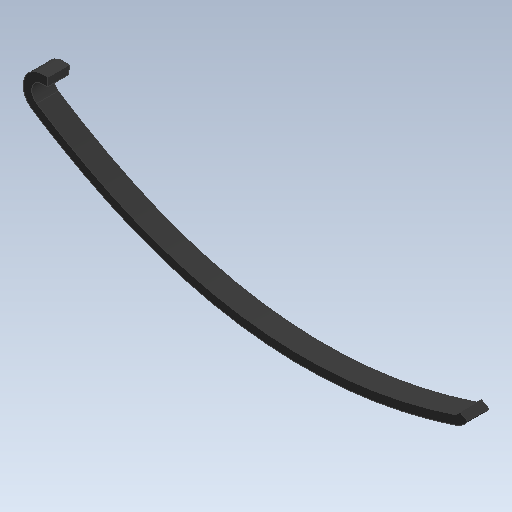
# Autodesk Inventor part: 脚ゴム
Saved by Autodesk Inventor 2020.2 (Build 242310000, 310)
## iProperties
Created: 2020-03-29
Part Number: 脚ゴム
Material: ゴム、シリコーン
Document SubType Name: Modeling
Designer: aoyama
Density: 1.25 g/cm^3
Appearance: ゴム - 黒
Mass: 1.4401 g
Surface Area: 16.3295 cm^2
Volume: 1.15208 cm^3
Author: aoyama
Autodesk Inventor part; units mm, degrees
ref_plane "YZ Plane" through (0, 0, 0) normal (1, 0, 0) x (0, 1, 0)
ref_plane "XZ Plane" through (0, 0, 0) normal (0, 1, 0) x (-1, 0, 0)
ref_plane "XY Plane" through (0, 0, 0) normal (0, 0, 1) x (1, 0, 0)
sketch "スケッチ1" plane through (0, 0, 0) normal (0, 0, 1) x (1, 0, 0)
  circle A0 centre (0, -30) radius 22.5
  arc A1 (33.5221, -76.1381) -> (34.7879, -75.2018) centre (32.744, -73.7622) ccw
  arc A2 (25.323, -41.3574) -> (34.2025, -71.7318) centre (49.1917, -50.8648) ccw
  arc A3 (25.323, -41.3574) -> (17.6049, -10.4152) centre (-0.0473, -31.252) ccw
  arc A4 (17.6049, -10.4152) -> (7.2408, -4.7162) centre (-0.2944, -30.6931) ccw
  arc A5 (5.1078, -1.4883) -> (7.2408, -4.7162) centre (8.0549, -1.8596) ccw
  arc A6 (5.1078, -1.4883) -> (-5.8369, -1.4852) centre (-0.3643, -0.7018) ccw
  arc A7 (-5.8369, -1.4852) -> (-5.7215, -2.051) centre (-0.3936, -0.6703) ccw
  arc A8 (-7.4636, -3.4089) -> (-5.7215, -2.051) centre (-8.3074, -0.53) ccw
  arc A9 (-7.4636, -3.4089) -> (-26.8108, -27.5489) centre (0.1311, -29.3188) ccw
  arc A10 (-61.6776, -57.4439) -> (-26.8108, -27.5489) centre (-58.8657, -25.4432) ccw
  arc A11 (-61.6776, -57.4439) -> (-63.2531, -62.0341) centre (-61.8964, -59.9343) ccw
  spline S0 degree 4 poles (-63.2531, -62.0341) (-62.8771, -62.2771) (-62.3536, -62.6129) (-61.6848, -63.0378) (-60.873, -63.5467) (-60.2895, -63.9093) (-59.7104, -64.266) (-59.1355, -64.6169) (-58.5645, -64.9622) (-57.9972, -65.3021) (-57.4335, -65.6368) (-56.873, -65.9663) (-56.3156, -66.2909) (-55.7612, -66.6107) (-55.2095, -66.9258) (-54.6604, -67.2364) (-54.1137, -67.5424) (-53.5693, -67.8442) (-53.027, -68.1416) (-52.4867, -68.4349) (-51.9483, -68.7242) (-51.4116, -69.0094) (-50.8766, -69.2907) (-50.3432, -69.5682) (-49.8111, -69.8419) (-49.2804, -70.1119) (-48.7509, -70.3783) (-48.2225, -70.6411) (-47.6953, -70.9003) (-47.169, -71.156) (-46.6436, -71.4083) (-46.119, -71.6572) (-45.5953, -71.9028) (-45.0722, -72.145) (-44.5498, -72.384) (-44.0279, -72.6197) (-43.5066, -72.8522) (-42.9857, -73.0816) (-42.4653, -73.3077) (-41.9453, -73.5308) (-41.4255, -73.7507) (-40.9061, -73.9676) (-40.3869, -74.1814) (-39.868, -74.3922) (-39.3492, -74.5999) (-38.8305, -74.8047) (-38.312, -75.0064) (-37.7935, -75.2052) (-37.2751, -75.401) (-36.7567, -75.5939) (-36.2383, -75.7839) (-35.7198, -75.9709) (-35.2014, -76.155) (-34.6828, -76.3362) (-34.1642, -76.5146) (-33.6454, -76.69) (-33.1265, -76.8625) (-32.6075, -77.0322) (-32.0883, -77.199) (-31.5689, -77.363) (-31.0494, -77.5241) (-30.5297, -77.6823) (-30.0097, -77.8377) (-29.4895, -77.9902) (-28.9692, -78.1399) (-28.4485, -78.2868) (-27.9276, -78.4308) (-27.4065, -78.572) (-26.8851, -78.7103) (-26.3635, -78.8459) (-25.8416, -78.9785) (-25.3194, -79.1084) (-24.797, -79.2354) (-24.2743, -79.3596) (-23.7513, -79.481) (-23.228, -79.5995) (-22.7044, -79.7153) (-22.1806, -79.8281) (-21.6564, -79.9382) (-21.132, -80.0454) (-20.6073, -80.1498) (-20.0824, -80.2514) (-19.5571, -80.3501) (-19.0316, -80.446) (-18.5058, -80.5391) (-17.9797, -80.6294) (-17.4533, -80.7168) (-16.9267, -80.8014) (-16.3998, -80.8831) (-15.8727, -80.962) (-15.3453, -81.0381) (-14.8176, -81.1114) (-14.2897, -81.1818) (-13.7615, -81.2494) (-13.2331, -81.3141) (-12.7045, -81.376) (-12.1756, -81.4351) (-11.6464, -81.4913) (-11.1171, -81.5447) (-10.5875, -81.5953) (-10.0577, -81.643) (-9.5277, -81.6879) (-8.9975, -81.7299) (-8.467, -81.7691) (-7.9364, -81.8055) (-7.4055, -81.839) (-6.8745, -81.8697) (-6.3432, -81.8975) (-5.8118, -81.9225) (-5.2802, -81.9447) (-4.7483, -81.964) (-4.2163, -81.9805) (-3.6842, -81.9941) (-3.1518, -82.005) (-2.6192, -82.0129) (-2.0865, -82.0181) (-1.5536, -82.0204) (-1.0205, -82.0198) (-0.4873, -82.0165) (0.0461, -82.0103) (0.5798, -82.0012) (1.1136, -81.9893) (1.6475, -81.9746) (2.1817, -81.9571) (2.716, -81.9367) (3.2506, -81.9135) (3.7853, -81.8874) (4.3203, -81.8585) (4.8554, -81.8268) (5.3907, -81.7923) (5.9263, -81.7549) (6.4621, -81.7146) (6.9982, -81.6716) (7.5345, -81.6257) (8.071, -81.5769) (8.6078, -81.5254) (9.1449, -81.4709) (9.6823, -81.4137) (10.22, -81.3536) (10.758, -81.2906) (11.2964, -81.2248) (11.8351, -81.1561) (12.3742, -81.0846) (12.9137, -81.0102) (13.4537, -80.933) (13.9941, -80.8528) (14.5349, -80.7698) (15.0763, -80.6839) (15.6182, -80.5952) (16.1606, -80.5035) (16.7036, -80.4089) (17.2473, -80.3114) (17.7916, -80.211) (18.3366, -80.1077) (18.8824, -80.0014) (19.4289, -79.8921) (19.9763, -79.7799) (20.5245, -79.6647) (21.0736, -79.5465) (21.6238, -79.4253) (22.1749, -79.301) (22.7271, -79.1737) (23.2805, -79.0433) (23.835, -78.9099) (24.3908, -78.7733) (24.948, -78.6336) (25.5066, -78.4907) (26.0666, -78.3446) (26.6283, -78.1953) (27.1915, -78.0427) (27.7565, -77.8868) (28.3233, -77.7276) (28.8921, -77.5651) (29.4629, -77.3991) (30.0358, -77.2297) (30.6109, -77.0568) (31.1884, -76.8803) (31.9873, -76.6323) (32.6434, -76.4238) (33.1553, -76.2582) (33.5221, -76.1381) knots 0 0 0 0 0 0.015592 0.021777 0.027929 0.034049 0.040138 0.046199 0.052232 0.058238 0.064219 0.070176 0.076109 0.08202 0.08791 0.093779 0.099629 0.105459 0.111272 0.117067 0.122846 0.128609 0.134356 0.140089 0.145808 0.151513 0.157206 0.162886 0.168554 0.17421 0.179856 0.185491 0.191116 0.196731 0.202337 0.207934 0.213522 0.219102 0.224675 0.230239 0.235796 0.241346 0.246889 0.252426 0.257957 0.263481 0.269 0.274513 0.280021 0.285523 0.291021 0.296514 0.302002 0.307486 0.312966 0.318442 0.323914 0.329382 0.334846 0.340307 0.345765 0.351219 0.356671 0.362119 0.367565 0.373008 0.378448 0.383886 0.389321 0.394754 0.400185 0.405614 0.41104 0.416465 0.421888 0.427309 0.432729 0.438147 0.443563 0.448978 0.454391 0.459803 0.465214 0.470624 0.476032 0.48144 0.486846 0.492252 0.497656 0.50306 0.508463 0.513865 0.519267 0.524668 0.530069 0.535469 0.540869 0.546268 0.551667 0.557066 0.562465 0.567863 0.573262 0.57866 0.584059 0.589457 0.594856 0.600255 0.605655 0.611054 0.616454 0.621855 0.627256 0.632658 0.63806 0.643464 0.648868 0.654273 0.659678 0.665086 0.670494 0.675903 0.681314 0.686726 0.69214 0.697555 0.702972 0.708391 0.713811 0.719234 0.724659 0.730086 0.735515 0.740947 0.746382 0.751819 0.757259 0.762702 0.768149 0.773599 0.779052 0.784509 0.789969 0.795434 0.800903 0.806376 0.811854 0.817337 0.822825 0.828317 0.833816 0.83932 0.84483 0.850346 0.855869 0.861399 0.866935 0.872479 0.878031 0.883591 0.889159 0.894736 0.900321 0.905917 0.911522 0.917137 0.922763 0.9284 0.934049 0.93971 0.945383 0.951069 0.956769 0.962483 0.968212 0.973956 0.979716 0.985493 1 1 1 1 1
  arc A12 (34.1445, -78.0387) -> (35.3693, -70.1074) centre (32.744, -73.7622) ccw
  arc A13 (27.181, -42.0975) -> (35.3693, -70.1074) centre (49.1917, -50.8648) ccw
  arc A14 (27.181, -42.0975) -> (18.9132, -8.9024) centre (-0.0473, -31.252) ccw
  arc A15 (18.9132, -8.9024) -> (7.7922, -2.7937) centre (-0.2944, -30.6931) ccw
  arc A16 (7.0908, -1.7497) -> (7.7922, -2.7937) centre (8.0549, -1.8596) ccw
  arc A17 (7.0908, -1.7497) -> (-7.8158, -1.7749) centre (-0.3643, -0.7018) ccw
  arc A18 (-7.8158, -1.7749) -> (-7.8596, -1.4241) centre (-0.3936, -0.6703) ccw
  arc A19 (-8.0261, -1.4896) -> (-7.8596, -1.4241) centre (-8.3074, -0.53) ccw
  arc A20 (-8.0261, -1.4896) -> (-28.8065, -27.4178) centre (0.1311, -29.3188) ccw
  arc A21 (-61.5025, -55.4515) -> (-28.8065, -27.4178) centre (-58.8657, -25.4432) ccw
  arc A22 (-61.5025, -55.4515) -> (-64.3384, -63.714) centre (-61.8964, -59.9343) ccw
  line L0 (32.744, -73.7622) -> (36.7043, -75.899)
  line L1 (-58.8657, -25.4432) -> (-60.8013, -57.5088)
  line L2 (-61.8964, -59.9343) -> (-65.1475, -63.0456)
  line L3 (-61.8964, -59.9343) -> (-65.7346, -57.5851)
  line L4 (49.1917, -50.8648) -> (30.5824, -70.5938)
  arc A23 (-5.8375, -1.4811) -> (-5.8362, -1.4893) centre (-4.7979, -1.3331) ccw
  arc A24 (-5.8362, -1.4893) -> (-5.8121, -1.6365) centre (-0.3936, -0.6703) ccw
  arc A25 (-6.0587, -2.5158) -> (-5.8121, -1.6365) centre (-6.8458, -1.8208) ccw
  arc A26 (-7.4636, -3.4089) -> (-6.0587, -2.5158) centre (-8.3074, -0.53) ccw
  arc A27 (-7.4636, -3.4089) -> (-26.8108, -27.5489) centre (0.1311, -29.3188) ccw
  arc A28 (-61.6776, -57.4439) -> (-26.8108, -27.5489) centre (-58.8657, -25.4432) ccw
  arc A29 (-61.6776, -57.4439) -> (-63.2531, -62.0341) centre (-61.8964, -59.9343) ccw
  spline S1 degree 4 poles (-63.2531, -62.0341) (-62.8771, -62.2771) (-62.3536, -62.6129) (-61.6848, -63.0378) (-60.873, -63.5467) (-60.2895, -63.9093) (-59.7104, -64.266) (-59.1355, -64.6169) (-58.5645, -64.9622) (-57.9972, -65.3021) (-57.4335, -65.6368) (-56.873, -65.9663) (-56.3156, -66.2909) (-55.7612, -66.6107) (-55.2095, -66.9258) (-54.6604, -67.2364) (-54.1137, -67.5424) (-53.5693, -67.8442) (-53.027, -68.1416) (-52.4867, -68.4349) (-51.9483, -68.7242) (-51.4116, -69.0094) (-50.8766, -69.2907) (-50.3432, -69.5682) (-49.8111, -69.8419) (-49.2804, -70.1119) (-48.7509, -70.3783) (-48.2225, -70.6411) (-47.6953, -70.9003) (-47.169, -71.156) (-46.6436, -71.4083) (-46.119, -71.6572) (-45.5953, -71.9028) (-45.0722, -72.145) (-44.5498, -72.384) (-44.0279, -72.6197) (-43.5066, -72.8522) (-42.9857, -73.0816) (-42.4653, -73.3077) (-41.9453, -73.5308) (-41.4255, -73.7507) (-40.9061, -73.9676) (-40.3869, -74.1814) (-39.868, -74.3922) (-39.3492, -74.5999) (-38.8305, -74.8047) (-38.312, -75.0064) (-37.7935, -75.2052) (-37.2751, -75.401) (-36.7567, -75.5939) (-36.2383, -75.7839) (-35.7198, -75.9709) (-35.2014, -76.155) (-34.6828, -76.3362) (-34.1642, -76.5146) (-33.6454, -76.69) (-33.1265, -76.8625) (-32.6075, -77.0322) (-32.0883, -77.199) (-31.5689, -77.363) (-31.0494, -77.5241) (-30.5297, -77.6823) (-30.0097, -77.8377) (-29.4895, -77.9902) (-28.9692, -78.1399) (-28.4485, -78.2868) (-27.9276, -78.4308) (-27.4065, -78.572) (-26.8851, -78.7103) (-26.3635, -78.8459) (-25.8416, -78.9785) (-25.3194, -79.1084) (-24.797, -79.2354) (-24.2743, -79.3596) (-23.7513, -79.481) (-23.228, -79.5995) (-22.7044, -79.7153) (-22.1806, -79.8281) (-21.6564, -79.9382) (-21.132, -80.0454) (-20.6073, -80.1498) (-20.0824, -80.2514) (-19.5571, -80.3501) (-19.0316, -80.446) (-18.5058, -80.5391) (-17.9797, -80.6294) (-17.4533, -80.7168) (-16.9267, -80.8014) (-16.3998, -80.8831) (-15.8727, -80.962) (-15.3453, -81.0381) (-14.8176, -81.1114) (-14.2897, -81.1818) (-13.7615, -81.2494) (-13.2331, -81.3141) (-12.7045, -81.376) (-12.1756, -81.4351) (-11.6464, -81.4913) (-11.1171, -81.5447) (-10.5875, -81.5953) (-10.0577, -81.643) (-9.5277, -81.6879) (-8.9975, -81.7299) (-8.467, -81.7691) (-7.9364, -81.8055) (-7.4055, -81.839) (-6.8745, -81.8697) (-6.3432, -81.8975) (-5.8118, -81.9225) (-5.2802, -81.9447) (-4.7483, -81.964) (-4.2163, -81.9805) (-3.6842, -81.9941) (-3.1518, -82.005) (-2.6192, -82.0129) (-2.0865, -82.0181) (-1.5536, -82.0204) (-1.0205, -82.0198) (-0.4873, -82.0165) (0.0461, -82.0103) (0.5798, -82.0012) (1.1136, -81.9893) (1.6475, -81.9746) (2.1817, -81.9571) (2.716, -81.9367) (3.2506, -81.9135) (3.7853, -81.8874) (4.3203, -81.8585) (4.8554, -81.8268) (5.3907, -81.7923) (5.9263, -81.7549) (6.4621, -81.7146) (6.9982, -81.6716) (7.5345, -81.6257) (8.071, -81.5769) (8.6078, -81.5254) (9.1449, -81.4709) (9.6823, -81.4137) (10.22, -81.3536) (10.758, -81.2906) (11.2964, -81.2248) (11.8351, -81.1561) (12.3742, -81.0846) (12.9137, -81.0102) (13.4537, -80.933) (13.9941, -80.8528) (14.5349, -80.7698) (15.0763, -80.6839) (15.6182, -80.5952) (16.1606, -80.5035) (16.7036, -80.4089) (17.2473, -80.3114) (17.7916, -80.211) (18.3366, -80.1077) (18.8824, -80.0014) (19.4289, -79.8921) (19.9763, -79.7799) (20.5245, -79.6647) (21.0736, -79.5465) (21.6238, -79.4253) (22.1749, -79.301) (22.7271, -79.1737) (23.2805, -79.0433) (23.835, -78.9099) (24.3908, -78.7733) (24.948, -78.6336) (25.5066, -78.4907) (26.0666, -78.3446) (26.6283, -78.1953) (27.1915, -78.0427) (27.7565, -77.8868) (28.3233, -77.7276) (28.8921, -77.5651) (29.4629, -77.3991) (30.0358, -77.2297) (30.6109, -77.0568) (31.1884, -76.8803) (31.9873, -76.6323) (32.6434, -76.4238) (33.1553, -76.2582) (33.5221, -76.1381) knots 0 0 0 0 0 0.015592 0.021777 0.027929 0.034049 0.040138 0.046199 0.052232 0.058238 0.064219 0.070176 0.076109 0.08202 0.08791 0.093779 0.099629 0.105459 0.111272 0.117067 0.122846 0.128609 0.134356 0.140089 0.145808 0.151513 0.157206 0.162886 0.168554 0.17421 0.179856 0.185491 0.191116 0.196731 0.202337 0.207934 0.213522 0.219102 0.224675 0.230239 0.235796 0.241346 0.246889 0.252426 0.257957 0.263481 0.269 0.274513 0.280021 0.285523 0.291021 0.296514 0.302002 0.307486 0.312966 0.318442 0.323914 0.329382 0.334846 0.340307 0.345765 0.351219 0.356671 0.362119 0.367565 0.373008 0.378448 0.383886 0.389321 0.394754 0.400185 0.405614 0.41104 0.416465 0.421888 0.427309 0.432729 0.438147 0.443563 0.448978 0.454391 0.459803 0.465214 0.470624 0.476032 0.48144 0.486846 0.492252 0.497656 0.50306 0.508463 0.513865 0.519267 0.524668 0.530069 0.535469 0.540869 0.546268 0.551667 0.557066 0.562465 0.567863 0.573262 0.57866 0.584059 0.589457 0.594856 0.600255 0.605655 0.611054 0.616454 0.621855 0.627256 0.632658 0.63806 0.643464 0.648868 0.654273 0.659678 0.665086 0.670494 0.675903 0.681314 0.686726 0.69214 0.697555 0.702972 0.708391 0.713811 0.719234 0.724659 0.730086 0.735515 0.740947 0.746382 0.751819 0.757259 0.762702 0.768149 0.773599 0.779052 0.784509 0.789969 0.795434 0.800903 0.806376 0.811854 0.817337 0.822825 0.828317 0.833816 0.83932 0.84483 0.850346 0.855869 0.861399 0.866935 0.872479 0.878031 0.883591 0.889159 0.894736 0.900321 0.905917 0.911522 0.917137 0.922763 0.9284 0.934049 0.93971 0.945383 0.951069 0.956769 0.962483 0.968212 0.973956 0.979716 0.985493 1 1 1 1 1
  arc A30 (33.5221, -76.1381) -> (34.7879, -75.2018) centre (32.744, -73.7622) ccw
  arc A31 (34.7879, -75.2018) -> (34.2598, -73.0105) centre (33.5615, -74.3381) ccw
  arc A32 (25.323, -41.3574) -> (30.5824, -70.5938) centre (44.8156, -52.9421) ccw
  arc A33 (25.323, -41.3574) -> (17.6049, -10.4152) centre (-0.0473, -31.252) ccw
  arc A34 (17.6049, -10.4152) -> (7.2408, -4.7162) centre (-0.2944, -30.6931) ccw
  arc A35 (5.1078, -1.4883) -> (7.2408, -4.7162) centre (8.0549, -1.8596) ccw
  arc A36 (5.1078, -1.4883) -> (-5.8375, -1.4811) centre (-0.3643, -0.7018) ccw
  circle A37 centre (0, -30) radius 22.7
  arc A38 (30.5824, -70.5938) -> (34.2598, -73.0105) centre (44.8156, -52.9421) ccw
  arc A39 (34.7879, -75.2018) -> (34.2025, -71.7318) centre (32.744, -73.7622) ccw
  arc A40 (31.8378, -69.0369) -> (35.1909, -71.2404) centre (44.8156, -52.9421) ccw
  arc A41 (36.423, -76.3535) -> (35.1909, -71.2404) centre (33.5615, -74.3381) ccw
  spline S2 degree 5 poles (-64.3384, -63.714) (-58.3884, -67.5577) (-52.2614, -71.1261) (-45.9065, -74.3086) (-33.0908, -79.5522) (-19.6141, -82.7098) (-12.9369, -83.7013) (0.6571, -84.5608) (14.2099, -83.176) (20.9822, -81.9204) (27.6266, -80.1731) (34.1445, -78.0387) knots 0 0 0 0 0 0 0.342867 0.342867 0.342867 0.668023 0.668023 0.668023 1 1 1 1 1 1
  point P0 (0, 0)
  point P1 (0, 0)
  point P2 (34.9441, -74.9493)
  point P3 (-60.6808, -55.5124)
  point P4 (-63.7026, -61.6628)
  point P5 (-64.0288, -58.6292)
  point P6 (32.9348, -68.0999)
  point P7 (0, 0)
  point P8 (-5.8121, -1.6365)
  point P9 (25.323, -41.3574)
  point P10 (-5.8121, -1.6365)
  point P11 (34.9441, -74.9493)
  point P12 (-63.7026, -61.6628)
  point P13 (25.323, -41.3574)
  point P14 (36.6963, -75.8947)
  point P15 (31.9593, -69.1341)
  point P16 (34.9338, -74.9438)
  dimension "d0" = 2
  dimension "d3" = 2
  constraints: 84 point on circle, 42 centre point, 10 end point, 1 concentric, 1 line through centre, 59 other
  measures "d3" radial gap between concentric circles of A40 A38
extrude "押し出し1" add sketch "スケッチ1" along normal blind 5 contours A10 A11 L3 A22 A21 L1 | A11 L2 A22 L3 | L0 A41 A12 S2 A22 L2 A11 S0 A1 A39 | L0 A12 A41
